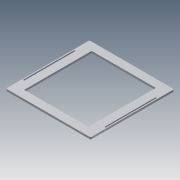
# Autodesk Inventor part: TopDiagonalPanel
Saved by Autodesk Inventor 2014 (Build 180170000, 170)
## iProperties
Created: 2014-08-11
Part Number: TopDiagonalPanel
Material: Generic
Document SubType Name: Modeling
Designer: Peele
Density: 1 g/cm^3
Appearance: White
Author: Peele
Autodesk Inventor part; units mm, degrees
ref_plane "YZ Plane" through (0, 0, 0) normal (1, 0, 0) x (0, 1, 0)
ref_plane "XZ Plane" through (0, 0, 0) normal (0, 1, 0) x (-1, 0, 0)
ref_plane "XY Plane" through (0, 0, 0) normal (0, 0, 1) x (1, 0, 0)
sketch "Sketch1" plane through (0, 0, 0) normal (0, 0, 1) x (1, 0, 0)
  line L0 (-132, -130.1931) -> (132, -130.1931)
  line L1 (132, -130.1931) -> (132, 130.1931)
  line L2 (132, 130.1931) -> (-132, 130.1931)
  line L3 (-132, 130.1931) -> (-132, -130.1931)
  line L4 (-132, -130.1931) -> (132, 130.1931) construction
  line L5 (132, -130.1931) -> (-132, 130.1931) construction
  point P0 (0, 0)
  dimension "d0" = 264
  dimension "d1" = 260.3863
  constraints: 12 end point, 2 midpoint, 2 parallel, 1 horizontal, 1 perpendicular
  measures "d0" distance of L0.start L0.end
  measures "d1" distance of L2.end L0.start
extrude "Extrusion1" add sketch "Sketch1" along normal blind 6
sketch "Sketch2" plane through (0, 0, 6) normal (0, 0, 1) x (1, 0, 0)
  line L0 (-132, -130.1931) -> (132, -130.1931) projected
  line L1 (132, 130.1931) -> (-132, 130.1931) projected
  line L2 (-132, 130.1931) -> (-132, -130.1931) projected
  line L3 (-129, 80.1931) -> (-125, 80.1931)
  line L4 (-125, 80.1931) -> (-125, -80.1931)
  line L5 (-125, -80.1931) -> (-129, -80.1931)
  line L6 (-129, -80.1931) -> (-129, 80.1931)
  line L7 (-129, 80.1931) -> (-125, -80.1931) construction
  line L8 (-125, 80.1931) -> (-129, -80.1931) construction
  point P0 (0, 0)
  point P1 (-127, 0)
  dimension "d5" = 3
  dimension "d6" = 4
  dimension "d7" = 50
  dimension "d101" = 50
  constraints: 12 end point, 2 midpoint, 2 parallel, 1 horizontal, 1 perpendicular
  measures "d5" distance between parallel lines of L2 L6
  measures "d6" distance of L3.start L3.end
  measures "d7" distance between parallel lines of L1 L3
  measures "d101" distance between parallel lines of L5 L0
extrude "Extrusion2" cut sketch "Sketch2" against normal through all
mirror "Mirror1" about plane through (0, 0, 0) normal (1, 0, 0) of "Extrusion2"
fillet "Fillet1" radius 3 4 edges at (132, 130.1931, 3) (132, -130.1931, 3) (-132, 130.1931, 3) (-132, -130.1931, 3)
sketch "Sketch3" plane through (0, 0, 6) normal (0, 0, 1) x (1, 0, 0)
  line L0 (129, 130.1931) -> (-129, 130.1931) projected
  line L1 (-125, 80.1931) -> (-125, -80.1931) projected
  line L2 (-100, -105.1931) -> (100, -105.1931)
  line L3 (100, -105.1931) -> (100, 105.1931)
  line L4 (100, 105.1931) -> (-100, 105.1931)
  line L5 (-100, 105.1931) -> (-100, -105.1931)
  line L6 (-100, -105.1931) -> (100, 105.1931) construction
  line L7 (100, -105.1931) -> (-100, 105.1931) construction
  point P0 (0, 0)
  dimension "d12" = 25
  dimension "d13" = 25
  constraints: 12 end point, 2 midpoint, 2 parallel, 1 horizontal, 1 perpendicular
  measures "d12" distance between parallel lines of L0 L4
  measures "d13" distance between parallel lines of L1 L5
extrude "Extrusion3" cut sketch "Sketch3" against normal through all
body "Solid1"
